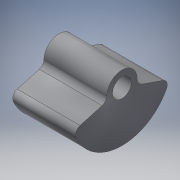
# Autodesk Inventor part: Cam
Saved by Autodesk Inventor 2016 (Build 200138000, 138)
## iProperties
Created: 2016-04-09
Part Number: Cam
Material: GFRC
Document SubType Name: Modeling
Designer: Vijay
Density: 1.7 g/cm^3
Appearance: Flat - Polished Gray
Author: Vijay
Autodesk Inventor part; units mm, degrees
ref_plane "YZ Plane" through (0, 0, 0) normal (1, 0, 0) x (0, 1, 0)
ref_plane "XZ Plane" through (0, 0, 0) normal (0, 1, 0) x (-1, 0, 0)
ref_plane "XY Plane" through (0, 0, 0) normal (0, 0, 1) x (1, 0, 0)
sketch "Sketch1" plane through (0, 0, 0) normal (1, 0, 0) x (0, 1, 0)
  arc A0 (-0.6481, 1.4629) -> (-0.7335, -1.422) centre (0, 0) ccw
  circle A1 centre (0, 0) radius 0.3
  arc A2 (-0.0182, -0.4866) -> (0.0106, 0.4868) centre (0, 0) ccw
  line L0 (-0.1776, 0.6327) -> (-0.3745, 1.3341)
  line L1 (-0.2147, -0.6211) -> (-0.4528, -1.3096)
  arc A3 (-0.0182, -0.4866) -> (-0.2147, -0.6211) centre (-0.0257, -0.6864) ccw
  arc A4 (-0.1776, 0.6327) -> (0.0106, 0.4868) centre (0.0149, 0.6867) ccw
  arc A5 (-0.3745, 1.3341) -> (-0.6481, 1.4629) centre (-0.5671, 1.28) ccw
  arc A6 (-0.7335, -1.422) -> (-0.4528, -1.3096) centre (-0.6418, -1.2442) ccw
  point P0 (-0.1464, 0.3788)
  point P1 (-0.4325, 1.5404)
  point P2 (-0.5229, -1.5122)
  point P3 (-0.1316, 0.4688)
  point P4 (-0.1591, -0.4602)
  dimension "d3" = 0.6
  dimension "d10" = 0.2
  constraints: 16 point on circle, 8 tangent, 7 centre point, 4 end point, 4 point on line, 3 equal radius, 2 coincident
  measures "d3" diameter of A1
  measures "d10" radius of A3
extrude "Extrusion1" add sketch "Sketch1" along normal blind 2
body "Solid1"
